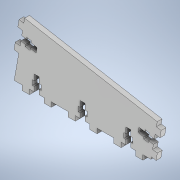
# Autodesk Inventor part: tc_support_down
Saved by Autodesk Inventor 2020.1 (Build 241239000, 239)
## iProperties
Created: 2019-07-16
Part Number: tc_support_down
Material: Acier inoxydable
Document SubType Name: Modeling
Designer: Thibault
Density: 8 g/cm^3
Appearance: Semi-poli
extra_height_front: 10,900 mm
extra_height_back: 1,008 mm
tc_base_support_dist: 56,100 mm
tc_anchor_dist: 19,100 mm
Author: Thibault
Autodesk Inventor part; units mm, degrees
ref_plane "YZ Plane" through (0, 0, 0) normal (1, 0, 0) x (0, 1, 0)
ref_plane "XZ Plane" through (0, 0, 0) normal (0, 1, 0) x (-1, 0, 0)
ref_plane "XY Plane" through (0, 0, 0) normal (0, 0, 1) x (1, 0, 0)
sketch "Anchor (screw side)" plane through (0, 0, 0) normal (0, 0, 1) x (1, 0, 0)
  circle A0 centre (93.8994, 50.3042) radius 1.05
  line L0 (90.8494, 51.3542) -> (87.7494, 51.3542)
  line L1 (87.7494, 51.3542) -> (87.7494, 49.2542)
  line L2 (87.7494, 49.2542) -> (90.8494, 49.2542)
  line L3 (90.8494, 49.2542) -> (90.8494, 51.3542)
  line L4 (100.0494, 51.3542) -> (96.9494, 51.3542)
  line L5 (96.9494, 51.3542) -> (96.9494, 49.2542)
  line L6 (96.9494, 49.2542) -> (100.0494, 49.2542)
  line L7 (100.0494, 49.2542) -> (100.0494, 51.3542)
  line L8 (90.8494, 51.3542) -> (96.9494, 49.2542) construction
  line L9 (96.9494, 51.3542) -> (90.8494, 49.2542) construction
  line L10 (85.7494, 53.3542) -> (102.0494, 53.3542) construction
  line L11 (102.0494, 53.3542) -> (102.0494, 47.2542) construction
  line L12 (102.0494, 47.2542) -> (85.7494, 47.2542) construction
  line L13 (85.7494, 47.2542) -> (85.7494, 53.3542) construction
  point P0 (103.5798, 50.1132)
  dimension "d27" = 2.1
  dimension "d28" = 3.1
  dimension "d29" = 2.1
  dimension "slot_distance" = 6.1
  dimension "d34" = 2
  dimension "d35" = 2
  dimension "d36" = 2
  dimension "d37" = 2
  measures "d27" diameter of A0
  measures "d28" distance of L2.end L1.end
  measures "d29" distance of L1.end L0.end
  measures "slot_distance" distance between parallel lines of L5 L3
  measures "d34" distance between parallel lines of L0 L10
  measures "d35" distance between parallel lines of L12 L2
  measures "d36" distance between parallel lines of L11 L7
  measures "d37" distance between parallel lines of L13 L1
sketch "Anchor (nut side)" plane through (0, 0, 0) normal (0, 0, 1) x (1, 0, 0)
  line L0 (11.1, 0) -> (9.1, 0)
  line L1 (9.1, 0) -> (9.1, -2)
  line L2 (9.1, -2) -> (9.9, -2)
  line L3 (9.9, -2) -> (9.9, -4)
  line L4 (6.2, -4) -> (6.2, -2)
  line L5 (6.2, -2) -> (7, -2)
  line L6 (7, -2) -> (7, 0)
  line L7 (7, 0) -> (5, 0)
  line L8 (2, 0) -> (2, 2)
  line L9 (2, 0) -> (3, 0) construction
  line L10 (2, 2) -> (5, 2)
  line L11 (5, 2) -> (5, 0)
  line L12 (11.1, 0) -> (11.1, 2)
  line L13 (11.1, 2) -> (14.1, 2)
  line L14 (14.1, 2) -> (14.1, 0)
  line L15 (0, 0) -> (2, 0)
  line L16 (14.1, 0) -> (16.1, 0)
  line L17 (6.2, -4) -> (7, -4)
  line L18 (9.9, -4) -> (9.1, -4)
  line L19 (7, -4) -> (7, -6.25)
  line L20 (9.1, -4) -> (9.1, -6.25)
  line L21 (7.25, -6.5) -> (8.05, -6.5)
  arc A0 (7, -6.25) -> (7.25, -6.5) centre (7.25, -6.25) ccw
  arc A1 (8.85, -6.5) -> (9.1, -6.25) centre (8.85, -6.25) ccw
  line L22 (8.05, -6.5) -> (8.85, -6.5)
  line L23 (8.05, -3.8983) -> (8.05, -9.959) construction
  point P0 (9.1321, -0.6227)
  point P1 (7, -6.5)
  point P2 (9.1, -6.5)
  dimension "d3" = 2
  dimension "d7" = 6.1
  dimension "d10" = 2
  dimension "d11" = 2
  dimension "d12" = 0.8
  dimension "d13" = 2
  dimension "d14" = 0.8
  dimension "d15" = 2.1
  dimension "d18" = 2
  dimension "d19" = 0.8
  dimension "d20" = 0.8
  dimension "d21" = 2.5
  dimension "d22" = 2.5
  dimension "d23" = 2.1
  dimension "d38" = 2
  dimension "d39" = 0.25
  dimension "d120" = 3
  measures "d3" distance of point (0, 0) L8.start
  measures "d7" distance of L7.end L0.start
  measures "d10" distance of L0.start L0.end
  measures "d11" distance of L0.end L1.end
  measures "d12" distance of L1.end L2.end
  measures "d13" distance of L2.end L3.end
  measures "d14" distance of L4.end L5.end
  measures "d15" distance of L6.end L0.end
  measures "d18" distance of L14.end point (16.1, 0)
  measures "d19" distance of L4.start L17.end
  measures "d20" distance of L3.end L18.end
  measures "d21" distance of L17.end point (7, -6.5)
  measures "d22" distance of L18.end point (9.1, -6.5)
  measures "d23" distance of L17.end L18.end
  measures "d38" distance of the line from the sketch origin of L10
  measures "d39" radius of A0
  measures "d120" distance of L8.end L10.end
derived "shared_parameters.ipt"
sketch "Esquisse2" plane through (0, 0, 0) normal (0, 0, 1) x (1, 0, 0)
  line L0 (-1.0016, 15.2398) -> (1.9984, 15.2398)
  line L1 (18.0984, 15.2398) -> (21.0984, 15.2398)
  line L2 (-17.1016, 15.2398) -> (-18.4343, 15.2398)
  line L3 (37.1984, 15.2398) -> (38.5311, 15.2398)
  line L4 (-18.4343, 15.2398) -> (-16.8888, 24.0046)
  line L5 (-14.0931, 39.86) -> (41.1546, 30.1184)
  line L6 (38.3589, 14.263) -> (38.5311, 15.2398)
  line L7 (-12.1016, 15.2398) -> (-10.1016, 15.2398)
  line L8 (-10.1016, 15.2398) -> (-10.1016, 17.2398)
  line L9 (-10.1016, 17.2398) -> (-10.9016, 17.2398)
  line L10 (-10.9016, 17.2398) -> (-10.9016, 19.2398)
  line L11 (-7.2016, 19.2398) -> (-7.2016, 17.2398)
  line L12 (-7.2016, 17.2398) -> (-8.0016, 17.2398)
  line L13 (-8.0016, 17.2398) -> (-8.0016, 15.2398)
  line L14 (-8.0016, 15.2398) -> (-6.0016, 15.2398)
  line L15 (-3.0016, 15.2398) -> (-3.0016, 13.2398)
  line L16 (-3.0016, 15.2398) -> (-4.0016, 15.2398) construction
  line L17 (-3.0016, 13.2398) -> (-6.0016, 13.2398)
  line L18 (-6.0016, 13.2398) -> (-6.0016, 15.2398)
  line L19 (-12.1016, 15.2398) -> (-12.1016, 13.2398)
  line L20 (-12.1016, 13.2398) -> (-15.1016, 13.2398)
  line L21 (-15.1016, 13.2398) -> (-15.1016, 15.2398)
  line L22 (-1.0016, 15.2398) -> (-3.0016, 15.2398)
  line L23 (-15.1016, 15.2398) -> (-17.1016, 15.2398)
  line L24 (-7.2016, 19.2398) -> (-8.0016, 19.2398)
  line L25 (-10.9016, 19.2398) -> (-10.1016, 19.2398)
  line L26 (-8.0016, 19.2398) -> (-8.0016, 21.4898)
  line L27 (-10.1016, 19.2398) -> (-10.1016, 21.4898)
  line L28 (-8.2516, 21.7398) -> (-9.0516, 21.7398)
  arc A0 (-8.0016, 21.4898) -> (-8.2516, 21.7398) centre (-8.2516, 21.4898) ccw
  arc A1 (-9.8516, 21.7398) -> (-10.1016, 21.4898) centre (-9.8516, 21.4898) ccw
  line L29 (-9.0516, 21.7398) -> (-9.8516, 21.7398)
  line L30 (-9.0516, 19.1381) -> (-9.0516, 25.1989) construction
  line L31 (6.9984, 15.2398) -> (8.9984, 15.2398)
  line L32 (8.9984, 15.2398) -> (8.9984, 17.2398)
  line L33 (8.9984, 17.2398) -> (8.1984, 17.2398)
  line L34 (8.1984, 17.2398) -> (8.1984, 19.2398)
  line L35 (11.8984, 19.2398) -> (11.8984, 17.2398)
  line L36 (11.8984, 17.2398) -> (11.0984, 17.2398)
  line L37 (11.0984, 17.2398) -> (11.0984, 15.2398)
  line L38 (11.0984, 15.2398) -> (13.0984, 15.2398)
  line L39 (16.0984, 15.2398) -> (16.0984, 13.2398)
  line L40 (16.0984, 15.2398) -> (15.0984, 15.2398) construction
  line L41 (16.0984, 13.2398) -> (13.0984, 13.2398)
  line L42 (13.0984, 13.2398) -> (13.0984, 15.2398)
  line L43 (6.9984, 15.2398) -> (6.9984, 13.2398)
  line L44 (6.9984, 13.2398) -> (3.9984, 13.2398)
  line L45 (3.9984, 13.2398) -> (3.9984, 15.2398)
  line L46 (18.0984, 15.2398) -> (16.0984, 15.2398)
  line L47 (3.9984, 15.2398) -> (1.9984, 15.2398)
  line L48 (11.8984, 19.2398) -> (11.0984, 19.2398)
  line L49 (8.1984, 19.2398) -> (8.9984, 19.2398)
  line L50 (11.0984, 19.2398) -> (11.0984, 21.4898)
  line L51 (8.9984, 19.2398) -> (8.9984, 21.4898)
  line L52 (10.8484, 21.7398) -> (10.0484, 21.7398)
  arc A2 (11.0984, 21.4898) -> (10.8484, 21.7398) centre (10.8484, 21.4898) ccw
  arc A3 (9.2484, 21.7398) -> (8.9984, 21.4898) centre (9.2484, 21.4898) ccw
  line L53 (10.0484, 21.7398) -> (9.2484, 21.7398)
  line L54 (10.0484, 19.1381) -> (10.0484, 25.1989) construction
  line L55 (26.0984, 15.2398) -> (28.0984, 15.2398)
  line L56 (28.0984, 15.2398) -> (28.0984, 17.2398)
  line L57 (28.0984, 17.2398) -> (27.2984, 17.2398)
  line L58 (27.2984, 17.2398) -> (27.2984, 19.2398)
  line L59 (30.9984, 19.2398) -> (30.9984, 17.2398)
  line L60 (30.9984, 17.2398) -> (30.1984, 17.2398)
  line L61 (30.1984, 17.2398) -> (30.1984, 15.2398)
  line L62 (30.1984, 15.2398) -> (32.1984, 15.2398)
  line L63 (35.1984, 15.2398) -> (35.1984, 13.2398)
  line L64 (35.1984, 15.2398) -> (34.1984, 15.2398) construction
  line L65 (35.1984, 13.2398) -> (32.1984, 13.2398)
  line L66 (32.1984, 13.2398) -> (32.1984, 15.2398)
  line L67 (26.0984, 15.2398) -> (26.0984, 13.2398)
  line L68 (26.0984, 13.2398) -> (23.0984, 13.2398)
  line L69 (23.0984, 13.2398) -> (23.0984, 15.2398)
  line L70 (37.1984, 15.2398) -> (35.1984, 15.2398)
  line L71 (23.0984, 15.2398) -> (21.0984, 15.2398)
  line L72 (30.9984, 19.2398) -> (30.1984, 19.2398)
  line L73 (27.2984, 19.2398) -> (28.0984, 19.2398)
  line L74 (30.1984, 19.2398) -> (30.1984, 21.4898)
  line L75 (28.0984, 19.2398) -> (28.0984, 21.4898)
  line L76 (29.9484, 21.7398) -> (29.1484, 21.7398)
  arc A4 (30.1984, 21.4898) -> (29.9484, 21.7398) centre (29.9484, 21.4898) ccw
  arc A5 (28.3484, 21.7398) -> (28.0984, 21.4898) centre (28.3484, 21.4898) ccw
  line L77 (29.1484, 21.7398) -> (28.3484, 21.7398)
  line L78 (29.1484, 19.1381) -> (29.1484, 25.1989) construction
  line L79 (-14.9613, 34.936) -> (-15.3086, 32.9664)
  line L80 (-15.3086, 32.9664) -> (-13.339, 32.6191)
  line L81 (-13.339, 32.6191) -> (-13.2001, 33.4069)
  line L82 (-13.2001, 33.4069) -> (-11.2305, 33.0596)
  line L83 (-11.873, 29.4158) -> (-13.8426, 29.7631)
  line L84 (-13.8426, 29.7631) -> (-13.7037, 30.551)
  line L85 (-13.7037, 30.551) -> (-15.6733, 30.8983)
  line L86 (-15.6733, 30.8983) -> (-16.0206, 28.9287)
  line L87 (-16.5415, 25.9742) -> (-18.5112, 26.3215)
  line L88 (-16.5415, 25.9742) -> (-16.3679, 26.9591) construction
  line L89 (-18.5112, 26.3215) -> (-17.9902, 29.276)
  line L90 (-17.9902, 29.276) -> (-16.0206, 28.9287)
  line L91 (-14.9613, 34.936) -> (-16.931, 35.2833)
  line L92 (-16.931, 35.2833) -> (-16.41, 38.2377)
  line L93 (-16.41, 38.2377) -> (-14.4404, 37.8904)
  line L94 (-16.8888, 24.0046) -> (-16.5415, 25.9742)
  line L95 (-14.4404, 37.8904) -> (-14.0931, 39.86)
  line L96 (-11.873, 29.4158) -> (-11.7341, 30.2037)
  line L97 (-11.2305, 33.0596) -> (-11.3694, 32.2718)
  line L98 (-11.7341, 30.2037) -> (-9.5183, 29.813)
  line L99 (-11.3694, 32.2718) -> (-9.1536, 31.8811)
  line L100 (-9.2286, 30.0158) -> (-9.0897, 30.8036)
  arc A6 (-9.5183, 29.813) -> (-9.2286, 30.0158) centre (-9.4748, 30.0592) ccw
  arc A7 (-8.9508, 31.5915) -> (-9.1536, 31.8811) centre (-9.197, 31.6349) ccw
  line L101 (-9.0897, 30.8036) -> (-8.9508, 31.5915)
  line L102 (-11.6519, 31.2554) -> (-5.6833, 30.203) construction
  line L103 (39.2271, 19.187) -> (39.5744, 21.1566)
  line L104 (39.5744, 21.1566) -> (37.6048, 21.5039)
  line L105 (37.6048, 21.5039) -> (37.4659, 20.7161)
  line L106 (37.4659, 20.7161) -> (35.4963, 21.0634)
  line L107 (36.1388, 24.7072) -> (38.1084, 24.3599)
  line L108 (38.1084, 24.3599) -> (37.9695, 23.572)
  line L109 (37.9695, 23.572) -> (39.9391, 23.2247)
  line L110 (39.9391, 23.2247) -> (40.2864, 25.1943)
  line L111 (40.8073, 28.1488) -> (42.7769, 27.8015)
  line L112 (40.8073, 28.1488) -> (40.6337, 27.1639) construction
  line L113 (42.7769, 27.8015) -> (42.256, 24.847)
  line L114 (42.256, 24.847) -> (40.2864, 25.1943)
  line L115 (39.2271, 19.187) -> (41.1967, 18.8397)
  line L116 (41.1967, 18.8397) -> (40.6758, 15.8853)
  line L117 (40.6758, 15.8853) -> (38.7062, 16.2326)
  line L118 (41.1546, 30.1184) -> (40.8073, 28.1488)
  line L119 (38.7062, 16.2326) -> (38.3589, 14.263)
  line L120 (36.1388, 24.7072) -> (35.9998, 23.9193)
  line L121 (35.4963, 21.0634) -> (35.6352, 21.8512)
  line L122 (35.9998, 23.9193) -> (33.784, 24.31)
  line L123 (35.6352, 21.8512) -> (33.4194, 22.2419)
  line L124 (33.4944, 24.1072) -> (33.3555, 23.3194)
  arc A8 (33.784, 24.31) -> (33.4944, 24.1072) centre (33.7406, 24.0638) ccw
  arc A9 (33.2166, 22.5315) -> (33.4194, 22.2419) centre (33.4628, 22.4881) ccw
  line L125 (33.3555, 23.3194) -> (33.2166, 22.5315)
  line L126 (35.9177, 22.8676) -> (29.949, 23.92) construction
  point P0 (0, 0)
  point P1 (-17.8871, 8.2607)
  point P2 (38.6612, 14.1706)
  point P3 (-17.9917, 8.6071)
  dimension "d1" = 7
  dimension "d2" = 7
  dimension "tc_anchor_dist" = 19.1
  dimension "height" = 25
  dimension "d41" = 56.1
  dimension "d44" = 80
  dimension "extra_height_front" = 10.9
  dimension "extra_height_back" = 1.0081
  constraints: 14 end point, 5 horizontal, 1 collinear, 14 other
  measures "d41" distance of L5.end L5.start
  measures "d44" angle of L2 L4
extrude "Extrusion1" add sketch "Esquisse2" along normal blind 2
equation "\"d41\" = tc_base_support_dist"
equation "\"d31\" = sheet_thickness"
equation "\"tc_base_support_dist\" = 56.1"
equation "\"sheet_thickness\" = 2"
